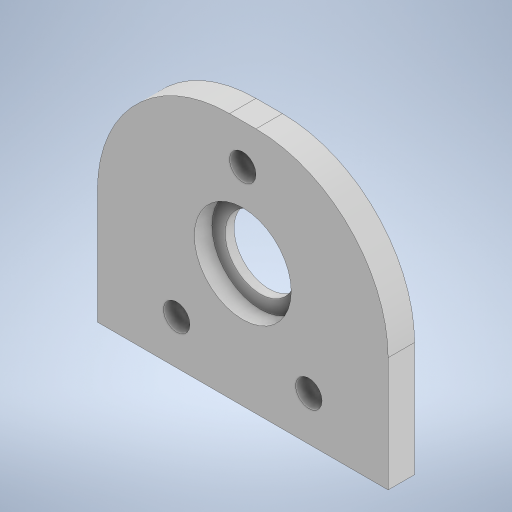
# Autodesk Inventor part: Arm6
Saved by Autodesk Inventor 2023 (Build 270158000, 158)
## iProperties
Created: 2024-02-06
Part Number: Arm6
Material: Generic
Document SubType Name: Modeling
Designer: victo
Density: 1 g/cm^3
Appearance: Default
Author: victo
Autodesk Inventor part; units mm, degrees
ref_plane "YZ Plane" through (0, 0, 0) normal (1, 0, 0) x (0, 1, 0)
ref_plane "XZ Plane" through (0, 0, 0) normal (0, 1, 0) x (-1, 0, 0)
ref_plane "XY Plane" through (0, 0, 0) normal (0, 0, 1) x (1, 0, 0)
sketch "Sketch1" plane through (0, 0, 0) normal (0, 0, 1) x (1, 0, 0)
  line L0 (0, 0) -> (33, 0)
  line L1 (33, 0) -> (33, 28)
  line L2 (33, 28) -> (0, 28)
  line L3 (0, 28) -> (0, 0)
  circle A0 centre (16.5, 14) radius 4
  circle A1 centre (16.5, 23.5) radius 1.5
  circle A2 centre (9, 5) radius 1.5
  circle A3 centre (24, 5) radius 1.5
  dimension "d0" = 33
  dimension "d1" = 28
  dimension "d2" = 8
  dimension "d3" = 14
  dimension "d4" = 16.5
  dimension "d5" = 3
  dimension "d6" = 3
  dimension "d7" = 3
  dimension "d8" = 4.5
  dimension "d9" = 0
  dimension "d10" = 15
  dimension "d11" = 5
  dimension "d12" = 9
  dimension "d13" = 5
  constraints: 8 end point, 4 centre point, 2 parallel, 1 horizontal, 1 perpendicular
  measures "d0" distance of L2.end L1.end
  measures "d1" distance of L1.end L0.end
  measures "d2" diameter of A0
  measures "d3" distance from line of L0 A0.centre
  measures "d4" distance from line of L3 A0.centre
  measures "d5" diameter of A1
  measures "d6" diameter of A2
  measures "d7" diameter of A3
  measures "d8" distance from line of L2 A1.centre
  measures "d9" horizontal distance of A1.centre A0.centre
  measures "d10" distance of A2.centre A3.centre
  measures "d11" distance from line of L0 A3.centre
  measures "d12" distance from line of L3 A2.centre
  measures "d13" distance from line of L0 A2.centre
extrude "Extrusion1" add sketch "Sketch1" along normal blind 3
sketch "Sketch2" plane through (0, 0, 3) normal (0, 0, 1) x (1, 0, 0)
  circle A0 centre (16.5, 14) radius 4 projected
  circle A1 centre (16.5, 14) radius 5.5
  point P0 (0, 0)
  dimension "d16" = 11
  constraints: 1 centre point, 1 coincident
  measures "d16" diameter of A1
extrude "Extrusion2" cut sketch "Sketch2" against normal blind 2 contours A0 | A1
fillet "Fillet1" radius 15 2 edges at (33, 28, 1.5) (0, 28, 1.5)
equation "\"d3\" = 0.5 * d1"
equation "\"d4\" = 0.5 * d0"
body "Solid1"
